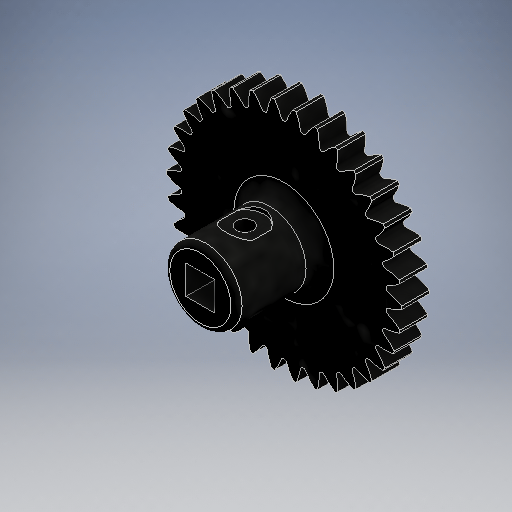
# Autodesk Inventor part: DriveGear2
Saved by Autodesk Inventor 2026.1 (Build 301233000, 233)
## iProperties
Created: 2025-09-07
Part Number: DriveGear2
Material: Plastic, Opaque Black
Document SubType Name: Modeling
Designer: Teddy
Density: 0.952 g/cm^3
Appearance: Smooth - Black
Author: Teddy
Autodesk Inventor part; units mm, degrees
ref_plane "YZ Plane" through (0, 0, 0) normal (1, 0, 0) x (0, 1, 0)
ref_plane "XZ Plane" through (0, 0, 0) normal (0, 1, 0) x (-1, 0, 0)
ref_plane "XY Plane" through (0, 0, 0) normal (0, 0, 1) x (1, 0, 0)
sketch "Sketch1" plane through (0, 0, 0) normal (0, 0, 1) x (1, 0, 0)
  spline S0 degree 3 poles (-2.1281, 26.8148) (-2.0309, 26.6746) (-1.8364, 26.3942) (-1.5663, 25.9593) (-1.3559, 25.5882) (-1.1984, 25.2855) (-1.0858, 25.0556) (-0.9794, 24.8229) (-0.8794, 24.5873) (-0.7872, 24.3486) (-0.7152, 24.1478) (-0.6661, 23.9844) (-0.6201, 23.8648) (-0.5684, 23.771) (-0.5175, 23.7025) (-0.4743, 23.6551) (-0.4264, 23.6126) (-0.3735, 23.5763) (-0.3155, 23.5488) (-0.2552, 23.5274) (-0.192, 23.5154) (-0.1066, 23.5143) (0, 23.5157) (0.1066, 23.5143) (0.192, 23.5154) (0.2552, 23.5274) (0.3155, 23.5488) (0.3735, 23.5763) (0.4264, 23.6126) (0.4743, 23.6551) (0.5175, 23.7025) (0.5684, 23.771) (0.6201, 23.8648) (0.6661, 23.9844) (0.7152, 24.1478) (0.7872, 24.3486) (0.8794, 24.5873) (0.9794, 24.8229) (1.0858, 25.0556) (1.1984, 25.2855) (1.3559, 25.5882) (1.5663, 25.9593) (1.8364, 26.3942) (2.0309, 26.6746) (2.1281, 26.8148) knots 0 0 0 0 0.051176 0.102352 0.153527 0.179117 0.204706 0.230295 0.255884 0.281473 0.307061 0.319857 0.332649 0.345435 0.351832 0.358226 0.364621 0.371019 0.37741 0.383798 0.390194 0.396593 0.409385 0.422178 0.428577 0.434973 0.441361 0.447752 0.45415 0.460545 0.466938 0.473335 0.486121 0.498914 0.511709 0.537298 0.562887 0.588476 0.614065 0.639654 0.665243 0.716418 0.767595 0.818771 0.818771 0.818771 0.818771
  circle A0 centre (0, 0) radius 23.5152 construction
  circle A1 centre (0, 0) radius 23.1108 construction
  circle A2 centre (0, 0) radius 25.5 construction
  circle A3 centre (0, 0) radius 26.8991
  point P0 (-1.84, 26.3918)
  point P1 (-1.5693, 25.9575)
  point P2 (-1.3174, 25.512)
  point P3 (-1.1993, 25.285)
  point P4 (-1.0869, 25.0552)
  point P5 (-0.9805, 24.8224)
  point P6 (-0.8807, 24.5868)
  point P7 (-0.7882, 24.3482)
  point P8 (-0.7036, 24.1067)
  point P9 (-0.6646, 23.9849)
  point P10 (-0.6174, 23.8659)
  point P11 (-0.5549, 23.7544)
  point P12 (-0.5166, 23.7031)
  point P13 (-0.4735, 23.6559)
  point P14 (-0.4256, 23.6136)
  point P15 (-0.3726, 23.5777)
  point P16 (-0.3151, 23.5498)
  point P17 (-0.2547, 23.529)
  point P18 (-0.1919, 23.5173)
  point P19 (-0.1279, 23.5148)
  point P20 (0, 23.5152)
  point P21 (0.1279, 23.5148)
  point P22 (0.1919, 23.5173)
  point P23 (0.2547, 23.529)
  point P24 (0.3151, 23.5498)
  point P25 (0.3726, 23.5777)
  point P26 (0.4256, 23.6136)
  point P27 (0.4735, 23.6559)
  point P28 (0.5166, 23.7031)
  point P29 (0.5549, 23.7544)
  point P30 (0.6174, 23.8659)
  point P31 (0.6646, 23.9849)
  point P32 (0.7036, 24.1067)
  point P33 (0.7882, 24.3482)
  point P34 (0.8807, 24.5868)
  point P35 (0.9805, 24.8224)
  point P36 (1.0869, 25.0552)
  point P37 (1.1993, 25.285)
  point P38 (1.3174, 25.512)
  point P39 (1.5693, 25.9575)
  point P40 (1.84, 26.3918)
  constraints: 4 centre point, 2 point on circle, 91 other
extrude "Extrusion1" add sketch "Sketch1" against normal blind 6.35
extrude "Extrusion2" cut sketch "Sketch1" against normal blind 25.4 contours A3 S0 picked at (-0.1026, 25.5483)
pattern_circular "Circular Pattern1" count 34 over 360 about axis through (0, 0, 0) along (0, 0, -1) of "Extrusion2"
sketch "Sketch2" plane through (0, 0, 0) normal (0, 0, 1) x (1, 0, 0)
  line L0 (-3.302, -3.302) -> (3.302, -3.302)
  line L1 (3.302, -3.302) -> (3.302, 3.302)
  line L2 (3.302, 3.302) -> (-3.302, 3.302)
  line L3 (-3.302, 3.302) -> (-3.302, -3.302)
  line L4 (-3.302, -3.302) -> (3.302, 3.302) construction
  line L5 (3.302, -3.302) -> (-3.302, 3.302) construction
  point P0 (0, 0)
  dimension "d7" = 6.604
  dimension "d8" = 6.604
  constraints: 12 end point, 2 midpoint, 2 parallel, 1 horizontal, 1 perpendicular
  measures "d7" distance of L0.end L1.end
  measures "d8" distance of L0.start L0.end
extrude "Extrusion3" cut sketch "Sketch2" against normal blind 25.4
sketch "Sketch3" plane through (0, 0, -6.35) normal (0, 0, -1) x (-1, 0, 0)
  circle A0 centre (0, 0) radius 8.255
  dimension "d11" = 16.51
  constraints: 1 centre point, 1 coincident
  measures "d11" diameter of A0
extrude "Extrusion4" cut sketch "Sketch3" against normal blind 5.08
sketch "Sketch4" plane through (0, 0, 0) normal (0, 0, 1) x (1, 0, 0)
  line L0 (-3.302, -3.302) -> (-3.302, 3.302) projected
  line L1 (-3.302, 3.302) -> (3.302, 3.302) projected
  line L2 (3.302, 3.302) -> (3.302, -3.302) projected
  line L3 (3.302, -3.302) -> (-3.302, -3.302) projected
  circle A0 centre (0, 0) radius 8.255
  constraints: 1 centre point, 1 coincident
extrude "Extrusion5" add sketch "Sketch4" along normal blind 19.05
fillet "Fillet1" radius 1.27 3 edges at (-8.255, 0, 19.05) (8.255, 0, -1.27) (8.255, 0, -6.35)
fillet "Fillet2" radius 3.175 1 edges at (-8.255, 0, 0)
sketch "Sketch5" plane through (-3.302, -3.302, -1.27) normal (0, 1, 0) x (1, 0, 0)
  circle A0 centre (3.302, -10.16) radius 1.905
  line L0 (6.604, -20.32) -> (0, -20.32) projected
  point P0 (3.302, -1.27)
  dimension "d18" = 3.81
  dimension "d19" = 10.16
  constraints: 1 centre point
  measures "d18" diameter of A0
  measures "d19" distance from line of L0 A0.centre
extrude "Extrusion6" cut sketch "Sketch5" along normal blind 19.05
ref_plane "Work Plane1" through (0, 8.255, 0) normal (0, -1, 0) x (1, 0, 0)
sketch "Sketch6" plane through (0, 8.255, 0) normal (0, -1, 0) x (1, 0, 0)
  circle A0 centre (0, 8.89) radius 1.905 projected
  circle A1 centre (0, 8.89) radius 4.445
  point P0 (0, 0)
  dimension "d22" = 8.89
  constraints: 1 centre point, 1 coincident
  measures "d22" diameter of A1
extrude "Extrusion7" cut sketch "Sketch6" along normal mid plane 1.905
equation "\"d0\" = FaceWidth"
equation "\"Module\" = 1.5"
equation "\"PressureAngle\" = 25deg"
equation "\"UnitProfileClearance\" = 0.157"
equation "\"UnitRoundRadius\" = 0.2245"
equation "\"HeadDiameter\" = 53.79818"
equation "\"RootDiameter\" = 47.03031"
equation "\"BaseDiameter\" = 46.2217"
equation "\"PitchDiameter\" = 51"
equation "\"FaceWidth\" = 6.35"
equation "\"HelixAngle\" = 0"
equation "\"UnitCorrection\" = -0.066059"
equation "\"UnitAddendumModification\" = 0.001214"
equation "\"CircularPitch\" = 4.71239"
equation "\"UnitBacklashShift\" = -0.100169"
equation "\"TotalToolShift\" = -0.24934"
equation "\"IsInternal\" = 0"
body "Solid1"
